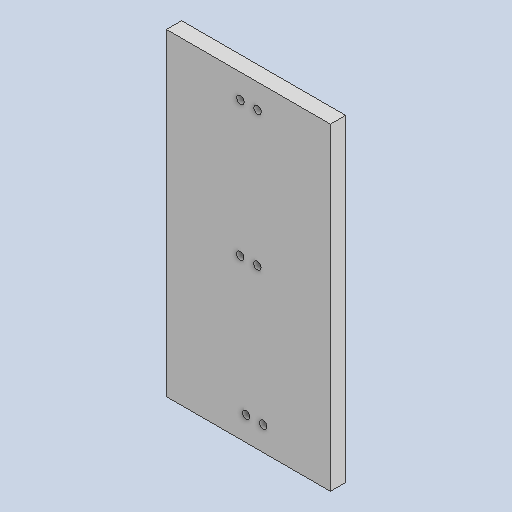
# Autodesk Inventor part: 0904_right_foot
Saved by Autodesk Inventor 2024.3 (Build 283343000, 343)
## iProperties
Created: 2024-09-04
Part Number: 0904_right_foot
Material: 일반
Document SubType Name: Modeling
Designer: gretc
Density: 1 g/cm^3
Appearance: 기본값
Author: gretc
Autodesk Inventor part; units mm, degrees
ref_plane "YZ Plane" through (0, 0, 0) normal (1, 0, 0) x (0, 1, 0)
ref_plane "XZ Plane" through (0, 0, 0) normal (0, 1, 0) x (-1, 0, 0)
ref_plane "XY Plane" through (0, 0, 0) normal (0, 0, 1) x (1, 0, 0)
ref_plane "작업 평면1" through (0, 0, 0) normal (0, 0, 1) x (1, 0, 0)
sketch "스케치1" plane through (0, 0, 0) normal (0, 0, 1) x (1, 0, 0)
  circle A0 centre (16.0813, 3) radius 1.5 projected
  circle A1 centre (9.3, 3) radius 1.5 projected
  ellipse E0 centre (18.3931, -50.3) end of major axis (18.3931, -51.8) minor radius 1.5 projected
  ellipse E1 centre (11.6071, -50.3) end of major axis (13.1071, -50.3) minor radius 1.5 projected
  ellipse E2 centre (16.1744, 56.34) end of major axis (16.1744, 57.84) minor radius 1.5 projected
  ellipse E3 centre (9.3931, 56.34) end of major axis (9.3931, 57.84) minor radius 1.5 projected
  line L0 (-19.8813, 65.8593) -> (-19.8813, -59.8593)
  line L1 (-19.8813, -59.8593) -> (44.9368, -59.8593)
  line L2 (44.9368, -59.8593) -> (44.9368, 65.8593)
  line L3 (44.9368, 65.8593) -> (-19.8813, 65.8593)
  line L4 (-19.8813, 65.8593) -> (44.9368, -59.8593) construction
  line L5 (-19.8813, -59.8593) -> (44.9368, 65.8593) construction
  point P0 (0, 0)
  point P1 (12.5278, 3)
  constraints: 12 end point, 2 midpoint, 2 parallel, 1 perpendicular, 1 vertical, 3 other
extrude "돌출1" add sketch "스케치1" along normal blind 6
